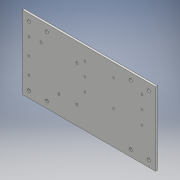
# Autodesk Inventor part: foot
Saved by Autodesk Inventor 2018 (Build 220112000, 112)
## iProperties
Created: 2018-11-26
Part Number: foot
Material: Generic
Document SubType Name: Modeling
Designer: bitbots
Density: 1 g/cm^3
Appearance: Default
Mass: 62.5233 g
Surface Area: 437.649 cm^2
Volume: 62.5233 cm^3
Author: bitbots
Autodesk Inventor part; units mm, degrees
ref_plane "YZ Plane" through (0, 0, 0) normal (1, 0, 0) x (0, 1, 0)
ref_plane "XZ Plane" through (0, 0, 0) normal (0, 1, 0) x (-1, 0, 0)
ref_plane "XY Plane" through (0, 0, 0) normal (0, 0, 1) x (1, 0, 0)
sketch "Sketch1" plane through (0, 0, 0) normal (0, 1, 0) x (-1, 0, 0)
  line L0 (-100, 55) -> (100, 55)
  line L1 (100, 55) -> (100, -55)
  line L2 (100, -55) -> (-100, -55)
  line L3 (-100, -55) -> (-100, 55)
  line L4 (-100, 55) -> (100, -55) construction
  line L5 (100, 55) -> (-100, -55) construction
  point P0 (0, 0)
  dimension "d0" = 200
  dimension "d1" = 110
  constraints: 12 end point, 2 midpoint, 2 parallel, 1 horizontal, 1 perpendicular
  measures "d0" distance of L1.end L2.end
  measures "d1" distance of L0.end L1.end
extrude "Extrusion1" add sketch "Sketch1" along normal blind 3
sketch "Sketch2" plane through (0, 3, 0) normal (0, 1, 0) x (1, 0, 0)
  line L0 (-100, -55) -> (100, -55) construction
  line L1 (100, -55) -> (100, -35) construction
  line L2 (100, -55) -> (100, 55) construction
  line L3 (100, -35) -> (80, -35) construction
  line L4 (80, -35) -> (37, -35) construction
  line L5 (80, -35) -> (123, -35) construction
  line L6 (37, -35) -> (-6, -35) construction
  line L7 (-6, -35) -> (-6, -15) construction
  line L8 (-6, -15) -> (-6, 5) construction
  line L9 (-6, 5) -> (37, 5) construction
  circle A0 centre (80, -35) radius 1.25
  circle A1 centre (37, -35) radius 1.25
  circle A2 centre (-6, -35) radius 1.25
  circle A3 centre (-6, -15) radius 1.25
  circle A4 centre (-6, 5) radius 1.25
  circle A5 centre (37, 5) radius 1.25
  line L10 (37, 5) -> (80, 5) construction
  line L11 (37, 5) -> (80, 5) construction
  line L12 (80, 5) -> (80, -15) construction
  circle A6 centre (80, 5) radius 1.25
  circle A7 centre (80, -15) radius 1.25
  point P0 (0, 0)
  dimension "d4" = 20
  dimension "d5" = 20
  dimension "d6" = 90
  dimension "d7" = 43
  dimension "d8" = 180
  dimension "d9" = 43
  dimension "d10" = 180
  dimension "d11" = 20
  dimension "d12" = 20
  dimension "d13" = 43
  dimension "d14" = 2.5
  dimension "d15" = 2.5
  dimension "d16" = 2.5
  dimension "d17" = 2.5
  dimension "d18" = 2.5
  dimension "d19" = 2.5
  dimension "d24" = 43
  dimension "d25" = 0
  dimension "d26" = 20
  dimension "d27" = 90
  dimension "d28" = 2.5
  dimension "d29" = 2.5
  constraints: 22 end point, 8 centre point, 8 coincident, 4 horizontal, 4 perpendicular, 3 collinear, 2 point on line
  measures "d4" distance of L0.end L1.end
  measures "d5" distance of L1.end L3.end
  measures "d6" angle of L3 L1
  measures "d7" distance of L3.end L4.end
  measures "d8" angle of L4 L5
  measures "d9" distance of L4.end L6.end
  measures "d10" angle of L6 L4
  measures "d11" distance of L6.end L7.end
  measures "d12" distance of L7.end L8.end
  measures "d13" distance of L8.end L9.end
  measures "d14" diameter of A0
  measures "d15" diameter of A1
  measures "d16" diameter of A2
  measures "d17" diameter of A3
  measures "d18" diameter of A4
  measures "d19" diameter of A5
  measures "d24" distance of L10.start L10.end
  measures "d25" distance between parallel lines of L10 L11
  measures "d26" distance of L10.end L12.end
  measures "d27" angle of L10 L12
  measures "d28" diameter of A6
  measures "d29" diameter of A7
extrude "Extrusion2" cut sketch "Sketch2" against normal blind 3
sketch "Sketch3" plane through (0, 3, 0) normal (0, 1, 0) x (1, 0, 0)
  line L0 (-100, -55) -> (-100, 55) construction
  line L1 (-100, -55) -> (-100, -45) construction
  line L2 (-100, -45) -> (-90, -45) construction
  circle A0 centre (-90, -45) radius 2.25
  line L3 (-90, -45) -> (-90, 45) construction
  line L4 (100, -55) -> (-100, -55) construction
  line L5 (-90, -45) -> (0, -45) construction
  line L6 (-90, 45) -> (90, 45) construction
  line L7 (90, 45) -> (90, -45) construction
  circle A1 centre (-90, 45) radius 2.25
  circle A2 centre (90, 45) radius 2.25
  circle A3 centre (90, -45) radius 2.25
  line L8 (90, -45) -> (63, -45) construction
  line L9 (-90, -45) -> (-63, -45) construction
  line L10 (-90, 45) -> (-63, 45) construction
  line L11 (90, 45) -> (63, 45) construction
  circle A4 centre (63, 45) radius 2.25
  circle A5 centre (63, -45) radius 2.25
  circle A6 centre (-63, -45) radius 2.25
  circle A7 centre (-63, 45) radius 2.25
  point P0 (0, 0)
  dimension "d32" = 10
  dimension "d33" = 10
  dimension "d34" = 4.5
  dimension "d35" = 90
  dimension "d36" = 90
  dimension "d37" = 180
  dimension "d38" = 90
  dimension "d39" = 90
  dimension "d40" = 4.5
  dimension "d41" = 4.5
  dimension "d42" = 4.5
  dimension "d45" = 27
  dimension "d46" = 27
  dimension "d47" = 4.5
  dimension "d48" = 4.5
  dimension "d49" = 4.5
  dimension "d50" = 4.5
  dimension "d64" = 27
  dimension "d65" = 27
  constraints: 20 end point, 8 centre point, 7 coincident, 5 point on line, 4 perpendicular, 2 horizontal, 1 vertical
  measures "d32" distance of L0.start L1.end
  measures "d33" distance of L1.end L2.end
  measures "d34" diameter of A0
  measures "d35" distance of L3.start L3.end
  measures "d36" angle of L5 L3
  measures "d37" distance of L3.end L6.end
  measures "d38" angle of L3 L6
  measures "d39" distance of L6.end L7.end
  measures "d40" diameter of A1
  measures "d41" diameter of A2
  measures "d42" diameter of A3
  measures "d45" distance of L8.start L8.end
  measures "d46" distance of L3.start L9.end
  measures "d47" diameter of A4
  measures "d48" diameter of A5
  measures "d49" diameter of A6
  measures "d50" diameter of A7
  measures "d64" distance of A7.centre L10.start
  measures "d65" distance of L11.start A4.centre
extrude "Extrusion4" cut sketch "Sketch3" against normal up to surface (3 mm away)
sketch "Sketch4" plane through (0, 0, 0) normal (0, -1, 0) x (1, 0, 0)
  circle A0 centre (-90, 45) radius 2.25 construction
  circle A1 centre (-63, 45) radius 2.25 construction
  circle A2 centre (-63, -45) radius 2.25 construction
  circle A3 centre (63, 45) radius 2.25 construction
  circle A4 centre (90, 45) radius 2.25 construction
  circle A5 centre (-90, -45) radius 2.25 construction
  circle A6 centre (-90, 45) radius 2.25 construction
  circle A7 centre (90, -45) radius 2.25 construction
  circle A8 centre (63, -45) radius 2.25 construction
  circle A9 centre (80, -5) radius 1.25 construction
  circle A10 centre (-6, -5) radius 1.25 construction
  circle A11 centre (-6, 35) radius 1.25 construction
  circle A12 centre (80, 35) radius 1.25 construction
  circle A13 centre (37, 35) radius 1.25 construction
  circle A14 centre (-6, 15) radius 1.25 construction
  circle A15 centre (37, -5) radius 1.25 construction
  circle A16 centre (80, 15) radius 1.25 construction
  line L0 (100, 55) -> (-100, 55) construction
  line L1 (-100, 55) -> (-100, -55) construction
  line L2 (-100, -55) -> (100, -55) construction
  line L3 (100, -55) -> (100, 55) construction
  circle A17 centre (-63, 45) radius 2.25 construction
  circle A18 centre (-63, -45) radius 2.25 construction
  circle A19 centre (63, 45) radius 2.25 construction
  circle A20 centre (90, 45) radius 2.25 construction
  circle A21 centre (-90, -45) radius 2.25 construction
  circle A22 centre (-90, 45) radius 2.25 construction
  circle A23 centre (90, -45) radius 2.25 construction
  circle A24 centre (63, -45) radius 2.25 construction
  circle A25 centre (80, -5) radius 1.25 construction
  circle A26 centre (-6, -5) radius 1.25 construction
  circle A27 centre (-6, 35) radius 1.25 construction
  circle A28 centre (80, 35) radius 1.25 construction
  circle A29 centre (37, 35) radius 1.25 construction
  circle A30 centre (-6, 15) radius 1.25 construction
  circle A31 centre (37, -5) radius 1.25 construction
  circle A32 centre (80, 15) radius 1.25 construction
  line L4 (100, 55) -> (-100, 55) construction
  line L5 (-100, 55) -> (-100, -55) construction
  line L6 (-100, -55) -> (100, -55) construction
  line L7 (100, -55) -> (100, 55) construction
  line L8 (-90, 45) -> (-90, 0) construction
  line L9 (-90, 45) -> (-45, 45) construction
  circle A33 centre (-90, 0) radius 1.25
  line L10 (-90, 0) -> (-90, 25) construction
  line L11 (-90, 0) -> (-90, -25) construction
  circle A34 centre (-90, 25) radius 1.25
  circle A35 centre (-90, -25) radius 1.25
  point P0 (0, 0)
  dimension "d55" = 45
  dimension "d56" = 90
  dimension "d57" = 2.5
  dimension "d58" = 25
  dimension "d59" = 25
  dimension "d60" = 2.5
  dimension "d61" = 2.5
  dimension "d90" = 10
  constraints: 8 end point, 3 centre point, 3 coincident, 2 point on line, 1 horizontal, 1 perpendicular, 1 vertical
  measures "d55" distance of L8.start L8.end
  measures "d56" angle of L8 L9
  measures "d57" diameter of A33
  measures "d58" distance of L10.start L10.end
  measures "d59" distance of L10.start L11.end
  measures "d60" diameter of A34
  measures "d61" diameter of A35
  measures "d90" distance from line of L5 L10.end
extrude "Extrusion5" cut sketch "Sketch4" against normal up to surface (3 mm away)
sketch "Sketch5" plane through (0, 3, 0) normal (0, 1, 0) x (1, 0, 0)
  line L0 (-100, -55) -> (100, -55) projected
  line L1 (-71.5, -55) -> (-43.5, -55) construction
  line L2 (-72, -27) -> (-72, 27)
  line L3 (-72, 27) -> (-45, 27)
  line L4 (-72, 27) -> (-45, 27) construction
  line L5 (-72, -27) -> (-18, -27)
  line L6 (-72, -27) -> (-18, -27) construction
  circle A0 centre (-72, -27) radius 1.5
  circle A1 centre (-18, -27) radius 1.5
  circle A2 centre (-45, 27) radius 1.5
  circle A3 centre (-90, -25) radius 1.25 projected
  circle A4 centre (-90, 25) radius 1.25 projected
  circle A5 centre (-90, 0) radius 1.25 projected
  circle A6 centre (-63, -45) radius 2.25 projected
  circle A7 centre (-63, 45) radius 2.25 projected
  circle A8 centre (63, -45) radius 2.25 projected
  circle A9 centre (90, -45) radius 2.25 projected
  circle A10 centre (-90, 45) radius 2.25 projected
  circle A11 centre (-90, -45) radius 2.25 projected
  circle A12 centre (90, 45) radius 2.25 projected
  circle A13 centre (63, 45) radius 2.25 projected
  circle A14 centre (80, 5) radius 1.25 projected
  circle A15 centre (-6, 5) radius 1.25 projected
  circle A16 centre (-6, -35) radius 1.25 projected
  circle A17 centre (80, -35) radius 1.25 projected
  circle A18 centre (37, -35) radius 1.25 projected
  circle A19 centre (-6, -15) radius 1.25 projected
  circle A20 centre (37, 5) radius 1.25 projected
  circle A21 centre (80, -15) radius 1.25 projected
  line L7 (-100, -55) -> (100, -55) projected
  line L8 (100, -55) -> (100, 55) projected
  line L9 (100, 55) -> (-100, 55) projected
  line L10 (-100, 55) -> (-100, -55) projected
  line L11 (-45, 27) -> (-18, 27)
  line L12 (-45, 27) -> (-18, 27) construction
  circle A22 centre (-18, 27) radius 1.5
  point P0 (0, 0)
  dimension "d70" = 54
  dimension "d72" = 27
  dimension "d73" = 0
  dimension "d74" = 54
  dimension "d75" = 0
  dimension "d76" = 3
  dimension "d77" = 3
  dimension "d79" = 3
  dimension "d82" = 12
  dimension "d83" = 28
  dimension "d84" = 90
  dimension "d85" = 27
  dimension "d86" = 0
  dimension "d87" = 3
  constraints: 16 end point, 7 horizontal, 4 centre point, 4 coincident, 3 collinear
  measures "d70" distance of L2.start L2.end
  measures "d72" distance of L2.end L3.end
  measures "d73" distance between parallel lines of L3 L4
  measures "d74" distance of L2.start L5.end
  measures "d75" distance between parallel lines of L5 L6
  measures "d76" diameter of A0
  measures "d77" diameter of A1
  measures "d79" diameter of A2
  measures "d82" horizontal distance of A1.centre A16.centre
  measures "d83" distance from line of L0 A1.centre
  measures "d84" angle of L5 L2
  measures "d85" distance of L11.start L11.end
  measures "d86" distance between parallel lines of L11 L12
  measures "d87" diameter of A22
extrude "Extrusion8" cut sketch "Sketch5" against normal blind 10 contours L5 A0 L2 | L2 A0 L5 | A22 | A2 L11 L3 | L3 L11 A2 | A1
body "Solid1"
